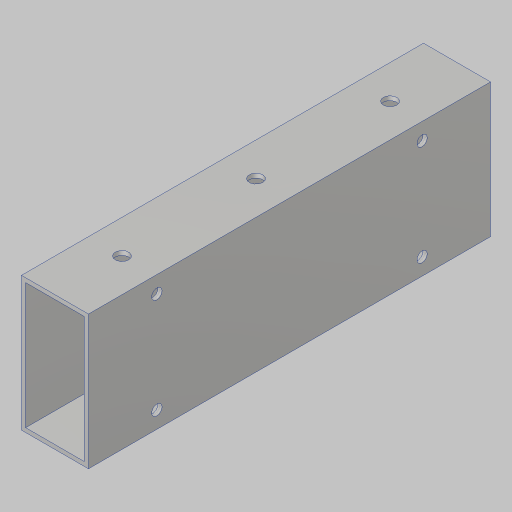
# Autodesk Inventor part: GP6-003
Saved by Autodesk Inventor 2023.5 (Build 275446000, 446)
## iProperties
RuleStatus: InUse
Created: 2025-02-23
Part Number: GP6-003
Material: Aluminum 6061
Document SubType Name: Modeling
Designer: slick
Mass: 304.185 g
Surface Area: 718.547 cm^2
Volume: 112.661 cm^3
Density: 2.7 g/cm^3
Appearance: Aluminum - Flat
AfterDocNew0: SHOW
AfterDocOpen0: SHOW
Author: slick
Autodesk Inventor part; units mm, degrees
ref_plane "YZ Plane" through (0, 0, 0) normal (1, 0, 0) x (0, 1, 0)
ref_plane "XZ Plane" through (0, 0, 0) normal (0, 1, 0) x (-1, 0, 0)
ref_plane "XY Plane" through (0, 0, 0) normal (0, 0, 1) x (1, 0, 0)
sketch "Sketch1" plane through (0, 0, 0) normal (0, 0, 1) x (1, 0, 0)
  line L0 (-12.7, -25.4) -> (12.7, -25.4)
  line L1 (12.7, -25.4) -> (12.7, 25.4)
  line L2 (12.7, 25.4) -> (-12.7, 25.4)
  line L3 (-12.7, 25.4) -> (-12.7, -25.4)
  line L4 (-12.7, -25.4) -> (12.7, 25.4) construction
  line L5 (12.7, -25.4) -> (-12.7, 25.4) construction
  line L6 (-11.1125, 23.8125) -> (11.1125, 23.8125)
  line L7 (11.1125, 23.8125) -> (11.1125, -23.8125)
  line L8 (11.1125, -23.8125) -> (-11.1125, -23.8125)
  line L9 (-11.1125, -23.8125) -> (-11.1125, 23.8125)
  point P0 (0, 0)
  dimension "width" = 25.4
  dimension "height" = 50.8
  dimension "thickness" = 1.5875
  constraints: 20 end point, 4 parallel, 2 midpoint, 2 perpendicular, 1 horizontal, 3 other
  measures "width" distance of L2.end L1.end
  measures "height" distance of L1.end L0.end
  measures "thickness" distance between parallel lines of L2 L6
extrude "Extrusion1" add sketch "Sketch1" along normal mid plane 152.4
sketch "Sketch2" plane through (-12.7, 25.4, 76.2) normal (0, 1, 0) x (1, 0, 0)
  line L0 (0, 152.4) -> (0, 0) construction
  line L1 (25.4, 0) -> (0, 0) construction
  line L2 (25.4, 152.4) -> (25.4, 0) construction
  line L3 (0, 152.4) -> (25.4, 152.4) construction
  line L4 (12.7, 127) -> (12.7, 25.4) construction
  point P0 (12.7, 76.2)
  point P1 (12.7, 76.2)
  point P2 (12.7, 76.2)
  dimension "d5" = 101.6
  constraints: 4 coincident, 2 end point, 1 midpoint, 1 vertical
  measures "d5" distance of L4.start L4.end
hole "Hole1" at (0, 25.4, -50.8) at (0, 25.4, 50.8) at (0, 25.4, 0) direction (0, -1, 0) diameter 5.1054 end through all clearance for "Flat Head Machine Screw (82)" size "#10" standard "Ansi Unified Screw Threads"
sketch "Sketch3" plane through (12.7, -25.4, 76.2) normal (1, 0, 0) x (0, 0, -1)
  line L0 (25.9391, 44.45) -> (126.4609, 44.45) construction
  line L1 (126.4609, 44.45) -> (126.4609, 6.35) construction
  line L2 (126.4609, 6.35) -> (25.9391, 6.35) construction
  line L3 (25.9391, 6.35) -> (25.9391, 44.45) construction
  line L4 (25.9391, 44.45) -> (126.4609, 6.35) construction
  line L5 (126.4609, 44.45) -> (25.9391, 6.35) construction
  circle A0 centre (76.2, 25.4) radius 60 construction
  circle A1 centre (76.2, 25.4) radius 47.5 construction
  circle A2 centre (76.2, 25.4) radius 53.75 construction
  dimension "d16" = 107.5
  dimension "d14" = 120
  dimension "d15" = 95
  dimension "d17" = 38.1
  constraints: 12 end point, 7 coincident, 2 centre point, 2 midpoint, 2 parallel, 1 horizontal, 1 perpendicular, 3 other
  measures "d14" diameter of A0
  measures "d15" diameter of A1
  measures "d17" distance of L2.end L0.start
hole "Hole2" at (12.7, 19.05, 50.2609) at (12.7, 19.05, -50.2609) at (12.7, -19.05, -50.2609) at (12.7, -19.05, 50.2609) direction (-1, 0, 0) diameter 3.9624 end through all thread size "10-32 UNF" class "2B" standard "ANSI Unified Screw Threads"
body "Solid1"
